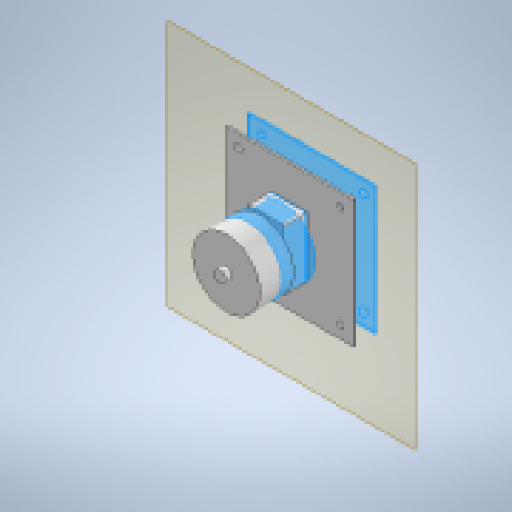
# Autodesk Inventor part: PCB_RW
Saved by Autodesk Inventor 2024 (Build 280153000, 153)
## iProperties
Created: 2023-06-28
Part Number: PCB_RW
Material: Genérico
Document SubType Name: Modeling
Designer: Personal
Density: 1 g/cm^3
Appearance: Valor por defecto
Author: Personal
Autodesk Inventor part; units mm, degrees
ref_plane "YZ Plane" through (0, 0, 0) normal (1, 0, 0) x (0, 1, 0)
ref_plane "XZ Plane" through (0, 0, 0) normal (0, 1, 0) x (-1, 0, 0)
ref_plane "XY Plane" through (0, 0, 0) normal (0, 0, 1) x (1, 0, 0)
ref_plane "Plano de trabajo1" through (0, 0, 0) normal (0, 0, 1) x (1, 0, 0)
sketch "Boceto1" plane through (0, 0, 0) normal (0, 0, 1) x (1, 0, 0)
  line L0 (50.85, -50.85) -> (50.85, 50.85) projected
  line L1 (50.85, 50.85) -> (-50.85, 50.85) projected
  line L2 (-50.85, 50.85) -> (-50.85, -50.85) projected
  line L3 (-50.85, -50.85) -> (50.85, -50.85) projected
  circle A0 centre (-40.8484, 40.8516) radius 2.8882 projected
  circle A1 centre (40.8516, 40.8516) radius 2.5 projected
  circle A2 centre (-40.8484, -40.8484) radius 2.8882 projected
  circle A3 centre (40.8516, -40.8484) radius 2.5 projected
  point P0 (0, 0)
extrude "Extrusión1" add sketch "Boceto1" along normal blind 1.65
sketch "Boceto2" plane through (0, 0, 1.65) normal (0, 0, 1) x (1, 0, 0)
  line L0 (14.2817, 24.0293) -> (-14.2817, 24.0293)
  line L1 (-14.2817, 24.0293) -> (-14.2817, -24.0293)
  line L2 (-14.2817, -24.0293) -> (14.2817, -24.0293)
  line L3 (14.2817, -24.0293) -> (14.2817, 24.0293)
  line L4 (14.2817, 24.0293) -> (-14.2817, -24.0293) construction
  line L5 (-14.2817, 24.0293) -> (14.2817, -24.0293) construction
  point P0 (0, 0)
  constraints: 12 end point, 2 midpoint, 2 parallel, 1 horizontal, 1 perpendicular
extrude "Extrusión2" add sketch "Boceto2" along normal blind 18.5
sketch "Boceto3" plane through (0, 0, 20.15) normal (0, 0, 1) x (1, 0, 0)
  circle A0 centre (0, 0) radius 4.3846
  constraints: 1 centre point, 1 coincident
extrude "Extrusión3" add sketch "Boceto3" along normal blind 5
sketch "Boceto4" plane through (0, 0, 25.15) normal (0, 0, 1) x (1, 0, 0)
  circle A0 centre (0, 0) radius 26.7
  dimension "d6" = 53.4
  constraints: 1 centre point, 1 coincident
  measures "d6" diameter of A0
extrude "Extrusión4" add sketch "Boceto4" along normal blind 27
sketch "Boceto5" plane through (0, 0, 52.15) normal (0, 0, 1) x (1, 0, 0)
  circle A0 centre (0, 0) radius 4.3846 projected
extrude "Extrusión5" add sketch "Boceto5" along normal blind 5
